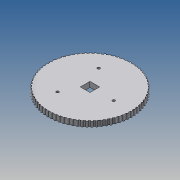
# Autodesk Inventor part: Plato Correa 2
Saved by Autodesk Inventor 2017 (Build 210142000, 142)
## iProperties
Part Number: Plato Correa 2
Material: Genérico
Document SubType Name: Modeling
Designer: FABLAB
Density: 1 g/cm^3
Appearance: Blanco
Author: FABLAB
Autodesk Inventor part; units mm, degrees
ref_plane "YZ Plane" through (0, 0, 0) normal (1, 0, 0) x (0, 1, 0)
ref_plane "XZ Plane" through (0, 0, 0) normal (0, 1, 0) x (-1, 0, 0)
ref_plane "XY Plane" through (0, 0, 0) normal (0, 0, 1) x (1, 0, 0)
sketch "Boceto1" plane through (0, 0, 0) normal (0, 0, 1) x (1, 0, 0)
  circle A0 centre (26.75, 0) radius 1.5 projected
  arc A1 (20.168, 17.783) -> (20.168, -17.783) centre (101.6471, 0) ccw construction
  arc A2 (5.3165, -26.3575) -> (20.168, -17.783) centre (11.375, -19.7021) ccw construction
  arc A3 (5.3165, -26.3575) -> (-25.4845, -8.5745) centre (-50.8235, -88.0289) ccw construction
  arc A4 (-25.4845, 8.5745) -> (-25.4845, -8.5745) centre (-22.75, 0) ccw construction
  arc A5 (-25.4845, 8.5745) -> (5.3165, 26.3575) centre (-50.8235, 88.0289) ccw construction
  arc A6 (20.168, 17.783) -> (5.3165, 26.3575) centre (11.375, 19.7021) ccw construction
  arc A7 (44.9403, -17.9838) -> (-44.9403, -17.9838) centre (0, 0) ccw construction
  circle A8 centre (-13.375, 23.1662) radius 1.5 projected
  circle A9 centre (-13.375, -23.1662) radius 1.5 projected
  circle A10 centre (45.905, 0) radius 1.1
  line L0 (0, 0) -> (0, -72) construction
  arc A11 (-20.105, -80.0454) -> (20.105, -80.0454) centre (0, -72) ccw construction
  line L1 (20.105, -80.0454) -> (44.9403, -17.9838) construction
  line L2 (-20.105, -80.0454) -> (-44.9403, -17.9838) construction
  circle A12 centre (45.7482, 3.7908) radius 1.1
  circle A13 centre (45.2789, 7.5557) radius 1.1
  circle A14 centre (44.5003, 11.269) radius 1.1
  circle A15 centre (43.4177, 14.9053) radius 1.1
  circle A16 centre (42.0386, 18.4398) radius 1.1
  circle A17 centre (40.3722, 21.8484) radius 1.1
  circle A18 centre (38.4301, 25.1077) radius 1.1
  circle A19 centre (36.2255, 28.1954) radius 1.1
  circle A20 centre (33.7734, 31.0906) radius 1.1
  circle A21 centre (31.0906, 33.7734) radius 1.1
  circle A22 centre (28.1954, 36.2255) radius 1.1
  circle A23 centre (25.1077, 38.4301) radius 1.1
  circle A24 centre (21.8484, 40.3722) radius 1.1
  circle A25 centre (18.4398, 42.0386) radius 1.1
  circle A26 centre (14.9053, 43.4177) radius 1.1
  circle A27 centre (11.269, 44.5003) radius 1.1
  circle A28 centre (7.5557, 45.2789) radius 1.1
  circle A29 centre (3.7908, 45.7482) radius 1.1
  circle A30 centre (0, 45.905) radius 1.1
  circle A31 centre (-3.7908, 45.7482) radius 1.1
  circle A32 centre (-7.5557, 45.2789) radius 1.1
  circle A33 centre (-11.269, 44.5003) radius 1.1
  circle A34 centre (-14.9053, 43.4177) radius 1.1
  circle A35 centre (-18.4398, 42.0386) radius 1.1
  circle A36 centre (-21.8484, 40.3722) radius 1.1
  circle A37 centre (-25.1077, 38.4301) radius 1.1
  circle A38 centre (-28.1954, 36.2255) radius 1.1
  circle A39 centre (-31.0906, 33.7734) radius 1.1
  circle A40 centre (-33.7734, 31.0906) radius 1.1
  circle A41 centre (-36.2255, 28.1954) radius 1.1
  circle A42 centre (-38.4301, 25.1077) radius 1.1
  circle A43 centre (-40.3722, 21.8484) radius 1.1
  circle A44 centre (-42.0386, 18.4398) radius 1.1
  circle A45 centre (-43.4177, 14.9053) radius 1.1
  circle A46 centre (-44.5003, 11.269) radius 1.1
  circle A47 centre (-45.2789, 7.5557) radius 1.1
  circle A48 centre (-45.7482, 3.7908) radius 1.1
  circle A49 centre (-45.905, 0) radius 1.1
  circle A50 centre (-45.7482, -3.7908) radius 1.1
  circle A51 centre (-45.2789, -7.5557) radius 1.1
  circle A52 centre (-44.5003, -11.269) radius 1.1
  circle A53 centre (-43.4177, -14.9053) radius 1.1
  circle A54 centre (-42.0386, -18.4398) radius 1.1
  circle A55 centre (-40.3722, -21.8484) radius 1.1
  circle A56 centre (-38.4301, -25.1077) radius 1.1
  circle A57 centre (-36.2255, -28.1954) radius 1.1
  circle A58 centre (-33.7734, -31.0906) radius 1.1
  circle A59 centre (-31.0906, -33.7734) radius 1.1
  circle A60 centre (-28.1954, -36.2255) radius 1.1
  circle A61 centre (-25.1077, -38.4301) radius 1.1
  circle A62 centre (-21.8484, -40.3722) radius 1.1
  circle A63 centre (-18.4398, -42.0386) radius 1.1
  circle A64 centre (-14.9053, -43.4177) radius 1.1
  circle A65 centre (-11.269, -44.5003) radius 1.1
  circle A66 centre (-7.5557, -45.2789) radius 1.1
  circle A67 centre (-3.7908, -45.7482) radius 1.1
  circle A68 centre (0, -45.905) radius 1.1
  circle A69 centre (3.7908, -45.7482) radius 1.1
  circle A70 centre (7.5557, -45.2789) radius 1.1
  circle A71 centre (11.269, -44.5003) radius 1.1
  circle A72 centre (14.9053, -43.4177) radius 1.1
  circle A73 centre (18.4398, -42.0386) radius 1.1
  arc A74 (-44.9403, -17.9838) -> (44.9403, -17.9838) centre (0, 0) ccw construction
  circle A75 centre (21.8484, -40.3722) radius 1.1
  circle A76 centre (0, 0) radius 45.905
  circle A77 centre (0, 0) radius 44.805 construction
  circle A78 centre (25.1077, -38.4301) radius 1.1
  circle A79 centre (28.1954, -36.2255) radius 1.1
  circle A80 centre (31.0906, -33.7734) radius 1.1
  circle A81 centre (33.7734, -31.0906) radius 1.1
  circle A82 centre (36.2255, -28.1954) radius 1.1
  circle A83 centre (38.4301, -25.1077) radius 1.1
  circle A84 centre (40.3722, -21.8484) radius 1.1
  circle A85 centre (42.0386, -18.4398) radius 1.1
  arc A86 (20.105, -80.0454) -> (-20.105, -80.0454) centre (0, -72) ccw construction
  circle A87 centre (43.4177, -14.9053) radius 1.1
  circle A88 centre (44.5003, -11.269) radius 1.1
  circle A89 centre (45.2789, -7.5557) radius 1.1
  line L3 (-7, -7) -> (7, -7)
  line L4 (7, -7) -> (7, 7)
  line L5 (7, 7) -> (-7, 7)
  line L6 (-7, 7) -> (-7, -7)
  circle A90 centre (0, 0) radius 72 construction
  circle A91 centre (45.7482, -3.7908) radius 1.1
  point P0 (0, -7)
  point P1 (-7, 0)
  dimension "d0" = 96.81
  dimension "d9" = 2.2
  dimension "d11" = 72
  dimension "d20" = 51.5451
  dimension "d21" = 188.9199
  dimension "d22" = 66.8464
  dimension "radio" = 21.655
  dimension "d26" = 360
  dimension "d28" = 3.794
  dimension "d31" = 3.6
  dimension "d32" = 2.5
  dimension "d33" = 14
  dimension "d34" = 84.5173
  constraints: 81 centre point, 14 end point, 8 point on circle, 8 tangent, 5 coincident, 3 horizontal alignment, 2 midpoint, 2 parallel, 2 perpendicular, 2 vertical alignment, 1 horizontal, 1 vertical, 157 other
  measures "d0" diameter of A7
  measures "d9" diameter of A10
  measures "d11" distance of L0.start L0.end
  measures "d22" distance of L1.start L1.end
  measures "radio" radius of A11
  measures "d28" distance of A18.centre A19.centre
  measures "d31" radial gap between concentric circles of A77 A7
  measures "d33" distance of L4.end L5.end
extrude "Extrusión1" add sketch "Boceto1" along normal blind 6
sketch "Boceto2" plane through (0, 0, 6) normal (0, 0, 1) x (1, 0, 0)
  circle A0 centre (0, 0) radius 41.5
  arc A1 (20.168, 17.783) -> (20.168, -17.783) centre (101.6471, 0) ccw
  arc A2 (20.168, 17.783) -> (5.3165, 26.3575) centre (11.375, 19.7021) ccw projected
  arc A3 (-25.4845, 8.5745) -> (5.3165, 26.3575) centre (-50.8235, 88.0289) ccw
  arc A4 (-25.4845, 8.5745) -> (-25.4845, -8.5745) centre (-22.75, 0) ccw
  arc A5 (5.3165, -26.3575) -> (-25.4845, -8.5745) centre (-50.8235, -88.0289) ccw projected
  arc A6 (5.3165, -26.3575) -> (20.168, -17.783) centre (11.375, -19.7021) ccw projected
  circle A7 centre (-13.375, -23.1662) radius 1.5 projected
  circle A8 centre (-13.375, 23.1662) radius 1.5 projected
  circle A9 centre (26.75, 0) radius 1.5 projected
  dimension "d30" = 83
  constraints: 6 point on circle, 4 centre point, 1 coincident, 11 other
  measures "d30" diameter of A0
sketch "Boceto3" plane through (0, 0, 0) normal (0, 0, -1) x (-1, 0, 0)
  circle A0 centre (0, 0) radius 41.5 projected
  circle A1 centre (0, 0) radius 36
  point P0 (0, 0)
  dimension "d6" = 5.5
  constraints: 1 centre point
  measures "d6" radial gap between concentric circles of A0 A1
